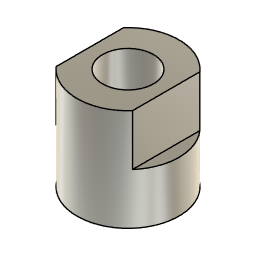
HIGH_ROD_END (Autodesk Fusion 360 design; units mm, degrees)
Autodesk Fusion 360 part; units mm, degrees
sketch "Esquisse1" plane through (0, 0, 0) normal (0, 0, 1) x (1, 0, 0)
  circle A0 centre (0, 0) radius 3
  circle A1 centre (0, 0) radius 6
  line L0 (-4.5, 8.8472) -> (4.5, 8.8472) construction
  line L1 (4.5, 8.8472) -> (4.5, -9.3481) construction
  line L2 (4.5, -9.3481) -> (-4.5, -9.3481) construction
  line L3 (-4.5, -9.3481) -> (-4.5, 8.8472) construction
  line L4 (4.5, 3.9686) -> (4.5, -3.9686)
  line L5 (-4.5, 3.9686) -> (-4.5, -3.9686)
  dimension "d1" = 6
  dimension "d2" = 12
  dimension "d3" = 9
  dimension "d4" = 4.5
  constraint coincident A0.centre A1.centre
  constraint horizontal L0
  constraint vertical L1
  constraint horizontal L2
  constraint vertical L3
  constraint coincident A1 L4.start
  constraint coincident L1 L4.start
  constraint coincident A1 L4.end
  constraint coincident L1 L4.end
  constraint coincident A1 L5.start
  constraint coincident L3 L5.start
  constraint coincident L3 L5.end
  constraint coincident A1 L5.end
  measures "d1" diameter of A0
  measures "d2" diameter of A1
  measures "d3" distance of L0.start L0.end
  measures "d4" distance of A0.centre L1
extrude "Extrusion3" add sketch "Esquisse1" along normal blind 12
sketch "Esquisse2" plane through (0, 0, 12) normal (0, 0, 1) x (-1, 0, 0)
  circle A0 centre (0, 0) radius 3
  circle A1 centre (0, 0) radius 6
  line L0 (4.5, -8.2141) -> (-4.5, -8.2141) construction
  line L1 (-4.5, -8.2141) -> (-4.5, 8.5) construction
  line L2 (-4.5, 8.5) -> (4.5, 8.5) construction
  line L3 (4.5, 8.5) -> (4.5, -8.2141) construction
  line L4 (4.5, 3.9686) -> (4.5, -3.9686)
  line L5 (-4.5, -3.9686) -> (-4.5, 3.9686)
  dimension "d12" = 9
  dimension "d13" = 4.5
  constraint horizontal L0
  constraint vertical L1
  constraint horizontal L2
  constraint vertical L3
  constraint coincident A1 L4.start
  constraint coincident L3 L4.start
  constraint coincident L3 L4.end
  constraint coincident A1 L4.end
  constraint coincident L1 L5.start
  constraint coincident A1 L5.start
  constraint coincident L1 L5.end
  constraint coincident A1 L5.end
  measures "d12" distance of L0.start L0.end
  measures "d13" distance of A0.centre L1
extrude "Extrusion4" cut sketch "Esquisse2" against normal blind 6 contours A1 L4 | A1 L5
